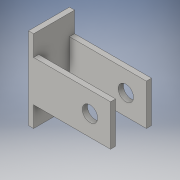
# Autodesk Inventor part: base
Saved by Autodesk Inventor 2016 (Build 200138000, 138)
## iProperties
Created: 2016-02-24
Part Number: base
Material: Generic
Document SubType Name: Modeling
Designer: gus
Density: 1 g/cm^3
Appearance: Default
Author: gus
Autodesk Inventor part; units mm, degrees
ref_plane "YZ Plane" through (0, 0, 0) normal (1, 0, 0) x (0, 1, 0)
ref_plane "XZ Plane" through (0, 0, 0) normal (0, 1, 0) x (-1, 0, 0)
ref_plane "XY Plane" through (0, 0, 0) normal (0, 0, 1) x (1, 0, 0)
sketch "Sketch1" plane through (0, 0, 0) normal (0, 1, 0) x (-1, 0, 0)
  line L0 (0, 0) -> (50.8, 0)
  line L1 (50.8, 0) -> (50.8, 25.4)
  line L2 (50.8, 25.4) -> (0, 25.4)
  line L3 (0, 25.4) -> (0, 22.225)
  line L4 (0, 22.225) -> (47.625, 22.225)
  line L5 (47.625, 22.225) -> (47.625, 3.175)
  line L6 (47.625, 3.175) -> (0, 3.175)
  line L7 (0, 3.175) -> (0, 0)
  dimension "d0" = 3.175
  dimension "d1" = 3.175
  dimension "d2" = 19.05
  dimension "d3" = 50.8
  constraints: 16 end point, 3 parallel, 3 perpendicular, 2 collinear, 1 horizontal, 1 point on line
  measures "d0" distance between parallel lines of L1 L5
  measures "d1" distance of L2.end L3.end
  measures "d2" distance of L4.end L5.end
  measures "d3" distance of L0.start L0.end
extrude "Extrusion1" add sketch "Sketch1" along normal blind 25.4
sketch "Sketch2" plane through (0, 25.4, 0) normal (0, 1, 0) x (1, 0, 0)
  line L0 (-50.8, -25.4) -> (0, -25.4) projected
  line L1 (-50.8, -25.4) -> (-47.625, -25.4)
  line L2 (-47.625, -25.4) -> (-47.625, 0)
  line L3 (-47.625, 0) -> (-50.8, 0)
  line L4 (-50.8, 0) -> (-50.8, -25.4)
  line L5 (-47.625, -22.225) -> (-47.625, -3.175) projected
  line L6 (0, 0) -> (-50.8, 0) projected
  constraints: 8 end point, 2 collinear, 2 parallel, 1 horizontal, 1 perpendicular
extrude "Extrusion2" add sketch "Sketch2" along normal blind 12.7
sketch "Sketch3" plane through (0, 0, 0) normal (0, -1, 0) x (1, 0, 0)
  line L0 (-50.8, 25.4) -> (0, 25.4) projected
  line L1 (0, 0) -> (-47.625, 0) projected
  line L2 (-50.8, 25.4) -> (-47.625, 25.4)
  line L3 (-47.625, 25.4) -> (-47.625, 0)
  line L4 (-47.625, 0) -> (-50.8, 0)
  line L5 (-50.8, 0) -> (-50.8, 25.4)
  constraints: 8 end point, 2 parallel, 1 horizontal, 1 perpendicular
extrude "Extrusion3" add sketch "Sketch3" along normal blind 12.7
sketch "Sketch4" plane through (-47.625, 0, 25.4) normal (0, 0, 1) x (1, 0, 0)
  circle A0 centre (34.925, 12.7) radius 4.7625
  line L0 (0, 0) -> (47.625, 0) projected
  line L1 (47.625, 0) -> (47.625, 25.4) projected
  dimension "d10" = 9.525
  dimension "d11" = 12.7
  dimension "d12" = 12.7
  constraints: 1 centre point
  measures "d10" diameter of A0
  measures "d11" distance from line of L0 A0.centre
  measures "d12" distance from line of L1 A0.centre
extrude "Extrusion4" cut sketch "Sketch4" against normal blind 25.4
body "Solid1"
